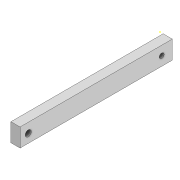
# Autodesk Inventor part: horizontal_strip
Saved by Autodesk Inventor 2021 (Build 250183000, 183)
## iProperties
Created: 2021-07-11
Part Number: horizontal_strip
Material: Generic
Document SubType Name: Modeling
Designer: Hp
Density: 1 g/cm^3
Appearance: Default
Author: Hp
Autodesk Inventor part; units mm, degrees
ref_plane "YZ Plane" through (0, 0, 0) normal (1, 0, 0) x (0, 1, 0)
ref_plane "XZ Plane" through (0, 0, 0) normal (0, 1, 0) x (-1, 0, 0)
ref_plane "XY Plane" through (0, 0, 0) normal (0, 0, 1) x (1, 0, 0)
sketch "Sketch1" plane through (0, 0, 0) normal (0, 0, 1) x (1, 0, 0)
  point P0 (0, 0)
sketch "Sketch2" plane through (0, 0, 0) normal (0, 0, 1) x (1, 0, 0)
  line L0 (20.3112, 0) -> (5.3112, 0)
  line L1 (5.3112, 0) -> (5.3112, -30)
  line L2 (5.3112, -30) -> (20.3112, -30)
  line L3 (20.3112, -30) -> (20.3112, 0)
  point P0 (0, 0)
  dimension "d0" = 15
  dimension "d1" = 30
  constraints: 8 end point, 2 parallel, 1 horizontal, 1 perpendicular
  measures "d0" distance of L2.end L1.end
  measures "d1" distance of L1.end L0.end
extrude "Extrusion1" add sketch "Sketch2" along normal blind 250
sketch "Sketch3" plane through (20.3112, -30, 0) normal (1, 0, 0) x (0, 0, -1)
  circle A0 centre (-17.4625, 15) radius 4
  point P0 (0, 30)
  dimension "d4" = 8
  constraints: 1 centre point
  measures "d4" diameter of A0
extrude "Extrusion2" cut sketch "Sketch3" against normal through all
sketch "Sketch4" plane through (20.3112, -30, 0) normal (1, 0, 0) x (0, 0, -1)
  circle A0 centre (-236.5375, 14.2875) radius 5
  point P0 (0, 30)
  dimension "d7" = 10
  constraints: 1 centre point
  measures "d7" diameter of A0
extrude "Extrusion3" cut sketch "Sketch4" against normal through all
body "Solid1"
